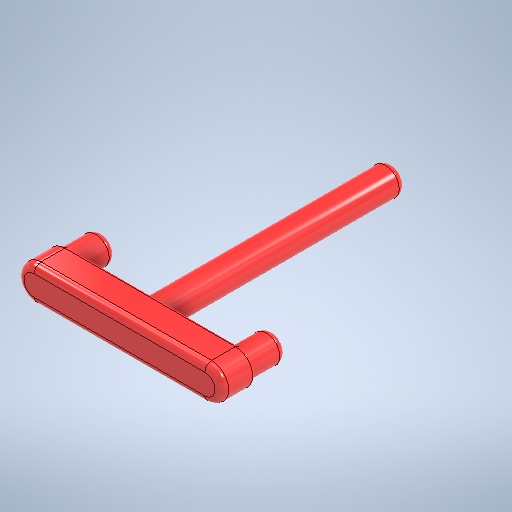
# Autodesk Inventor part: Steering Mounting Plate 3
Saved by Autodesk Inventor 2025.2 (Build 292293000, 293)
## iProperties
Created: 2025-03-15
Part Number: Steering Mounting Plate 3
Material: Generic
Document SubType Name: Modeling
Designer: eason
Density: 1 g/cm^3
Appearance: Light Red
Author: eason
Autodesk Inventor part; units mm, degrees
ref_plane "YZ Plane" through (0, 0, 0) normal (1, 0, 0) x (0, 1, 0)
ref_plane "XZ Plane" through (0, 0, 0) normal (0, 1, 0) x (-1, 0, 0)
ref_plane "XY Plane" through (0, 0, 0) normal (0, 0, 1) x (1, 0, 0)
sketch "Sketch1" plane through (0, 0, 0) normal (0, 0, 1) x (1, 0, 0)
  circle A0 centre (-12.5, 0) radius 2
  line L0 (0, -3.5) -> (0, 3.5) projected
  line L1 (-21, 0) -> (21, 0) projected
  arc A1 (-12.5, 2.5) -> (-12.5, -2.5) centre (-12.5, 0) ccw
  circle A2 centre (12.5, 0) radius 2
  arc A3 (12.5, -2.5) -> (12.5, 2.5) centre (12.5, 0) ccw
  line L2 (-12.5, 2.5) -> (12.5, 2.5)
  line L3 (-12.5, -2.5) -> (12.5, -2.5)
  point P0 (0, 0)
  dimension "d0" = 4
  dimension "d2" = 5
  dimension "d3" = 25
  constraints: 4 centre point, 4 end point, 4 point on circle, 2 coincident, 2 symmetric about line, 2 tangent, 1 horizontal, 1 parallel, 1 point on line, 2 other
  measures "d0" diameter of A0
  measures "d2" diameter of A1
  measures "d3" distance of A3.centre A0.centre
extrude "Extrusion1" add sketch "Sketch1" along normal blind 5
extrude "Extrusion2" add sketch "Sketch1" against normal blind 5 contours L1 A0 | A0 L1 | A2 L1 | L1 A2
sketch "Sketch2" plane through (0, 0, 0) normal (0, 0, -1) x (-1, 0, 0)
  circle A0 centre (0, 0) radius 2
  line L0 (0, -3.5996) -> (0, 4.0974) projected
  line L1 (21, 0) -> (-21, 0) projected
  dimension "d8" = 4
  constraints: 1 centre point, 1 midpoint, 1 point on line
  measures "d8" diameter of A0
extrude "Extrusion3" add sketch "Sketch2" along normal blind 35
fillet "Fillet1" radius 1 7 edges at (2, 0, -35) (10.5, 0, -5) (-14.5, 0, -5) (-15, 0, 5) (0, -2.5, 5) (15, 0, 5) (0, 2.5, 5)
fillet "Fillet2" radius 0.5 4 edges at (-15, 0, 0) (0, -2.5, 0) (15, 0, 0) (0, 2.5, 0)
body "Solid1"
